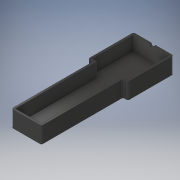
# Autodesk Inventor part: ajBottom
Saved by Autodesk Inventor 2018 (Build 220112000, 112)
## iProperties
Created: 2018-02-17
Part Number: ajBottom
Material: Generic
Document SubType Name: Modeling
Designer: artur
Density: 1 g/cm^3
Appearance: Default
Author: artur
Autodesk Inventor part; units mm, degrees
ref_plane "YZ Plane" through (0, 0, 0) normal (1, 0, 0) x (0, 1, 0)
ref_plane "XZ Plane" through (0, 0, 0) normal (0, 1, 0) x (-1, 0, 0)
ref_plane "XY Plane" through (0, 0, 0) normal (0, 0, 1) x (1, 0, 0)
sketch "Sketch1" plane through (0, 0, 0) normal (0, 1, 0) x (-1, 0, 0)
  line L0 (0, 0) -> (42, 0)
  line L1 (42, 0) -> (42, -115)
  line L2 (42, -115) -> (0, -115)
  line L3 (0, -115) -> (0, 0)
  line L4 (21, -115) -> (21, 0) construction
  line L5 (-7, -115) -> (49, -115)
  line L6 (49, -115) -> (49, -179)
  line L7 (49, -179) -> (-7, -179)
  line L8 (-7, -179) -> (-7, -115)
  line L9 (21, -179) -> (21, -115) construction
  dimension "d0" = 42
  dimension "d1" = 115
  dimension "d2" = 64
  dimension "d3" = 56
  constraints: 20 end point, 4 parallel, 3 midpoint, 2 collinear, 2 horizontal, 2 perpendicular, 1 coincident
  measures "d0" distance of L1.end L2.end
  measures "d1" distance of L0.end L1.end
  measures "d2" distance of L5.end L6.end
  measures "d3" distance of L6.end L7.end
extrude "Extrusion1" add sketch "Sketch1" along normal blind 23
shell "Shell1" thickness 2.54 removed faces 1 at (-14, 23, -38.3333)
fillet "Fillet1" radius 2 8 edges at (-42, 11.5, 0) (0, 11.5, 0) (0, 11.5, -115) (7, 11.5, -115) (-49, 11.5, -115) (-42, 11.5, -115) (7, 11.5, -179) (-49, 11.5, -179)
sketch "Sketch2" plane through (5, 0, -179) normal (0, 0, -1) x (-1, 0, 0)
  line L0 (51.46, 23) -> (0.54, 23) projected
  circle A0 centre (26, 23) radius 3.1
  line L1 (54, 0) -> (54, 23) projected
  line L2 (-2, 23) -> (-2, 0) projected
  point P0 (5, 0)
  dimension "d8" = 6.2
  dimension "d9" = 28
  dimension "d10" = 28
  constraints: 1 centre point, 1 midpoint
  measures "d8" diameter of A0
  measures "d9" distance from line of L1 A0.centre
  measures "d10" distance from line of A0.centre L2
extrude "Extrusion2" cut sketch "Sketch2" against normal blind 23
body "Solid1"
